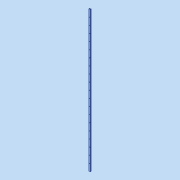
# Autodesk Inventor part: Prowadnica liniowa MGN9R 900mm
Saved by Autodesk Inventor 2018 (Build 220112000, 112)
## iProperties
Created: 2019-01-23
Part Number: Prowadnica liniowa MGN9R 900mm
Material: Ogólny
Document SubType Name: Modeling
Designer: Dawid
Density: 1 g/cm^3
Appearance: Aluminium — płaski
Author: Dawid
Autodesk Inventor part; units mm, degrees
ref_plane "YZ Plane" through (0, 0, 0) normal (1, 0, 0) x (0, 1, 0)
ref_plane "XZ Plane" through (0, 0, 0) normal (0, 1, 0) x (-1, 0, 0)
ref_plane "XY Plane" through (0, 0, 0) normal (0, 0, 1) x (1, 0, 0)
sketch "Szkic1" plane through (0, 0, 0) normal (0, 0, 1) x (1, 0, 0)
  line L0 (0, 0) -> (4.5, 0)
  line L1 (4.5, 6.5) -> (-4.5, 6.5)
  line L2 (-4.5, 0) -> (4.5, 0)
  line L3 (4.5, 6.5) -> (4.5, 5)
  line L4 (4.5, 5) -> (3, 5)
  line L5 (3, 5) -> (3, 3.5)
  line L6 (3, 3.5) -> (4.5, 3.5)
  line L7 (-4.5, 6.5) -> (-4.5, 5)
  line L8 (-4.5, 5) -> (-3, 5)
  line L9 (-3, 5) -> (-3, 3.5)
  line L10 (-3, 3.5) -> (-4.5, 3.5)
  line L11 (-4.5, 6.5) -> (-4.5, 5)
  line L12 (-4.5, 3.5) -> (-4.5, 0)
  line L13 (4.5, 0) -> (4.5, 3.5)
  line L14 (4.5, 5) -> (4.5, 6.5)
  dimension "d1" = 6.5
  dimension "d2" = 9
  dimension "d3" = 1.5
  dimension "d4" = 1.5
  dimension "d5" = 1.5
  dimension "d6" = 1.5
  dimension "d7" = 1.5
  dimension "d8" = 1.5
  constraints: 30 end point, 13 perpendicular, 1 collinear, 1 horizontal, 1 point on line, 1 vertical
  measures "d1" distance of L0.end L1.start
  measures "d2" distance of L1.start L1.end
  measures "d3" distance of L1.start L3.end
  measures "d4" distance of L3.end L4.end
  measures "d5" distance of L4.end L5.end
  measures "d6" distance of L1.end L7.end
  measures "d7" distance of L7.end L8.end
  measures "d8" distance of L8.end L9.end
extrude "Wyciągnięcie proste1" add sketch "Szkic1" along normal blind 900
sketch "Szkic2" plane through (-4.5, 6.5, 900) normal (0, 1, 0) x (1, 0, 0)
  line L0 (9, 900) -> (0, 900) projected
  line L1 (0, 900) -> (0, 0) projected
  line L2 (9, 0) -> (0, 0) projected
  line L3 (9, 900) -> (9, 0) projected
  line L4 (0, 0) -> (4.5, 0)
  line L5 (9, 0) -> (0, 0) projected
  line L6 (4.5, 0) -> (4.5, 900)
  line L7 (4.5, 900) -> (4.5, 855)
  circle A0 centre (4.5, 855) radius 1.75
  dimension "d11" = 4.5
  dimension "d12" = 45
  dimension "d13" = 3.5
  constraints: 6 end point, 1 centre point, 1 coincident, 1 midpoint, 1 perpendicular, 1 point on line
  measures "d11" distance of L1.end L4.end
  measures "d12" distance of L6.end L7.end
  measures "d13" diameter of A0
extrude "Wyciągnięcie proste2" cut sketch "Szkic2" against normal up to next contours A0 L6 | L6 A0
sketch "Szkic3" plane through (-4.5, 6.5, 900) normal (0, 1, 0) x (1, 0, 0)
  circle A0 centre (4.5, 855) radius 1.75 projected
  circle A1 centre (4.5, 855) radius 3
  point P0 (4.5, 900)
  dimension "d16" = 6
  constraints: 1 centre point, 1 coincident
  measures "d16" diameter of A1
extrude "Wyciągnięcie proste3" cut sketch "Szkic3" against normal blind 4
pattern_linear "Szyk prostokątny1" count 19 spacing 45 along (0, 0, 1) of "Wyciągnięcie proste3"
pattern_linear "Szyk prostokątny2" count 19 spacing 45 along (0, 0, 1) of "Wyciągnięcie proste2"
